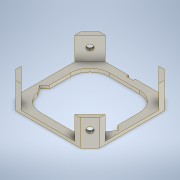
# Autodesk Inventor part: 로드셀 케이스2-3
Saved by Autodesk Inventor 2021 (Build 250183000, 183)
## iProperties
Created: 2021-08-10
Part Number: 로드셀 케이스2-3
Material: 티타늄
Document SubType Name: Modeling
Designer: Dongyoon
Density: 4.51 g/cm^3
Appearance: 티타늄
Author: Dongyoon
Autodesk Inventor part; units mm, degrees
ref_plane "YZ Plane" through (0, 0, 0) normal (1, 0, 0) x (0, 1, 0)
ref_plane "XZ Plane" through (0, 0, 0) normal (0, 1, 0) x (-1, 0, 0)
ref_plane "XY Plane" through (0, 0, 0) normal (0, 0, 1) x (1, 0, 0)
sketch "스케치1" plane through (0, 0, 0) normal (0, 1, 0) x (-1, 0, 0)
  line L0 (19.5, -19.5) -> (-19.5, -19.5)
  line L1 (-19.5, -19.5) -> (-19.5, 19.5)
  line L2 (-19.5, 19.5) -> (19.5, 19.5)
  line L3 (19.5, 19.5) -> (19.5, -19.5)
  line L4 (19.5, -19.5) -> (-19.5, 19.5) construction
  line L5 (-19.5, -19.5) -> (19.5, 19.5) construction
  line L6 (19.5, -12.5) -> (12.5, -19.5)
  line L7 (-12.5, -19.5) -> (-19.5, -12.5)
  line L8 (-19.5, 12.5) -> (-12.5, 19.5)
  line L9 (12.5, 19.5) -> (19.5, 12.5)
  line L10 (-15, -19.5) -> (-19.5, -15)
  line L11 (-19.5, 15) -> (-15, 19.5)
  line L12 (19.5, -15) -> (15, -19.5)
  line L13 (15, 19.5) -> (19.5, 15)
  point P0 (0, 0)
  dimension "d0" = 39
  dimension "d1" = 39
  dimension "d2" = 25
  dimension "d3" = 25
  dimension "d4" = 25
  dimension "d5" = 25
  dimension "d6" = 7
  dimension "d7" = 4.5
  dimension "d8" = 4.5
  dimension "d9" = 4.5
  dimension "d10" = 4.5
  dimension "d12" = 4.5
  dimension "d13" = 4.5
  dimension "d14" = 4.5
  constraints: 28 end point, 16 point on line, 4 perpendicular, 3 parallel, 2 midpoint, 1 horizontal
  measures "d0" distance of L1.end L2.end
  measures "d1" distance of L0.end L1.end
  measures "d2" distance of L7.start L6.end
  measures "d3" distance of L7.end L8.start
  measures "d4" distance of L9.start L8.end
  measures "d5" distance of L6.start L9.end
  measures "d6" horizontal distance of L7.start L7.end
  measures "d7" horizontal distance of L10.end L10.start
  measures "d8" horizontal distance of L10.start L10.end
  measures "d9" horizontal distance of L11.start L11.end
  measures "d10" horizontal distance of L11.start L11.end
  measures "d12" horizontal distance of L12.start L12.end
  measures "d13" horizontal distance of L13.start L13.end
  measures "d14" horizontal distance of L13.start L13.end
extrude "돌출1" add sketch "스케치1" along normal blind 1.5 contours L0 L7 L1 L8 L2 L9 L3 L6
extrude "돌출2" add sketch "스케치1" along normal blind 12.2 contours L0 L6 L3 L12 | L0 L10 L1 L7 | L9 L2 L13 L3 | L1 L11 L2 L8
sketch "스케치2" plane through (0, 1.5, 0) normal (0, 1, 0) x (1, 0, 0)
  line L0 (-7, 16) -> (7, 16)
  line L1 (16, 7) -> (16, -7)
  line L2 (7, -16) -> (-7, -16)
  line L3 (-16, -7) -> (-16, 7)
  arc A0 (-7, 16) -> (-16, 7) centre (-7, 7) ccw
  arc A1 (16, 7) -> (7, 16) centre (7, 7) ccw
  arc A2 (7, -16) -> (16, -7) centre (7, -7) ccw
  arc A3 (-16, -7) -> (-7, -16) centre (-7, -7) ccw
  line L4 (12.5, 19.5) -> (-12.5, 19.5) projected
  line L5 (19.5, -12.5) -> (19.5, 12.5) projected
  line L6 (-19.5, 12.5) -> (-19.5, -12.5) projected
  line L7 (-12.5, -19.5) -> (12.5, -19.5) projected
  point P0 (0, 0)
  dimension "d21" = 9
  dimension "d37" = 3.5
  dimension "d38" = 3.5
  dimension "d39" = 3.5
  dimension "d40" = 3.5
  constraints: 8 end point, 8 point on circle, 8 tangent, 4 centre point, 3 equal radius, 2 parallel, 1 horizontal, 1 perpendicular
  measures "d21" radius of A0
  measures "d37" distance between parallel lines of L4 L0
  measures "d38" distance between parallel lines of L5 L1
  measures "d39" distance between parallel lines of L6 L3
  measures "d40" distance between parallel lines of L2 L7
extrude "돌출3" cut sketch "스케치2" against normal through all
sketch "스케치3" plane through (15, 0, -19.5) normal (0.7071, 0, -0.7071) x (-0.7071, 0, -0.7071)
  line L0 (-6.364, 12.2) -> (0, 12.2) projected
  line L1 (-3.182, 12.2) -> (-3.182, 1.4483)
  circle A0 centre (-3.182, 7.2) radius 1.4
  dimension "d24" = 2.8
  dimension "d25" = 5
  constraints: 2 end point, 1 centre point, 1 midpoint, 1 point on line, 1 vertical
  measures "d24" diameter of A0
  measures "d25" distance from line of L0 A0.centre
extrude "돌출4" cut sketch "스케치3" against normal through all
mirror "미러1" about plane through (0, 0, 0) normal (0, 0, 1) of "돌출4"
sketch "스케치5" plane through (0, 1.5, 0) normal (0, 1, 0) x (1, 0, 0)
  line L0 (1.5, 18.5) -> (1.5, 20.3701)
  line L1 (1.5, 20.3701) -> (-1.4999, 20.3441)
  line L2 (-1.4999, 20.3441) -> (-1.4999, 18.5)
  line L3 (1.5, 18.5) -> (-1.4999, 18.5)
  line L4 (-7, 16) -> (7, 16) projected
  point P0 (0, 0)
  dimension "d31" = 3
  dimension "d32" = 1.5
  dimension "d48" = 2.5
  constraints: 8 end point, 1 parallel, 1 perpendicular, 1 vertical
  measures "d31" distance of L0.end L1.end
  measures "d32" distance from line of point (0, 0) L0
  measures "d48" distance between parallel lines of L4 L3
extrude "돌출5" cut sketch "스케치5" against normal blind 5
sketch "스케치6" plane through (0, 0, 0) normal (0, -1, 0) x (1, 0, 0)
  line L0 (-12.5, 19.5) -> (-19.5, 12.5) projected
  line L1 (16, -16) -> (-16, -16)
  line L2 (-16, -16) -> (-16, 16)
  line L3 (-16, 16) -> (16, 16)
  line L4 (16, 16) -> (16, -16)
  line L5 (16, -16) -> (-16, 16) construction
  line L6 (-16, -16) -> (16, 16) construction
  line L7 (10, 10) -> (-10, 10)
  line L8 (-10, 10) -> (-10, -10)
  line L9 (-10, -10) -> (10, -10)
  line L10 (10, -10) -> (10, 10)
  line L11 (18.2, 12.5) -> (18.2, 3)
  line L12 (19.5, 15) -> (19.5, -15) projected
  line L13 (6.886, 3) -> (18.2, 3)
  line L14 (6.886, 8.3) -> (16, 8.3)
  line L15 (6.886, 5.1) -> (18.2, 5.1)
  line L16 (16, 7) -> (16, -7) projected
  line L17 (16, 3) -> (18.2, 5.1)
  arc A0 (16, 7) -> (7, 16) centre (7, 7) ccw projected
  arc A1 (16, 7) -> (7, 16) centre (7, 7) ccw
  line L18 (18.2, 5.1) -> (16, 8.3)
  line L19 (15.8779, 8.4776) -> (16, 8.3)
  line L20 (0, 0) -> (0, 16)
  line L21 (-7, 16) -> (7, 16) projected
  line L22 (-16, 16) -> (-16, -16)
  line L23 (-16, 3) -> (-18.2, 5.1)
  arc A2 (-7, 16) -> (-16, 7) centre (-7, 7) ccw
  line L24 (-18.2, 5.1) -> (-16, 8.3)
  line L25 (-15.8779, 8.4776) -> (-16, 8.3)
  point P0 (16, 3)
  point P1 (-16, 7)
  dimension "d41" = 6
  dimension "d42" = 1.3
  dimension "d43" = 19
  dimension "d44" = 5.3
  dimension "d45" = 3.2
  constraints: 44 end point, 9 point on line, 7 symmetric about line, 6 point on circle, 5 parallel, 4 midpoint, 4 perpendicular, 2 centre point, 2 horizontal, 1 coincident, 1 vertical, 4 other
  measures "d41" distance between parallel lines of L3 L7
  measures "d42" distance between parallel lines of L11 L12
  measures "d43" distance between parallel lines of L1 L13
  measures "d44" distance between parallel lines of L13 L14
  measures "d45" distance between parallel lines of L14 L15
extrude "돌출6" cut sketch "스케치6" against normal blind 10 contours L23 L24 L2 | L4 L15 L17 | L2 L25 A2 | L4 L18 L15 | A0 L14 L4 | L14 A0 L19
